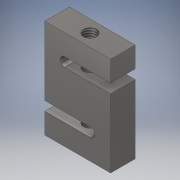
# Autodesk Inventor part: loadcell_s_500kg
Saved by Autodesk Inventor 2019.4 (Build 234330000, 330)
## iProperties
Created: 2020-09-27
Part Number: loadcell_s_500kg
Material: Stainless Steel
Document SubType Name: Modeling
Designer: deanv
Density: 8 g/cm^3
Appearance: Semi-Polished
Author: deanv
Autodesk Inventor part; units mm, degrees
ref_plane "YZ Plane" through (0, 0, 0) normal (1, 0, 0) x (0, 1, 0)
ref_plane "XZ Plane" through (0, 0, 0) normal (0, 1, 0) x (-1, 0, 0)
ref_plane "XY Plane" through (0, 0, 0) normal (0, 0, 1) x (1, 0, 0)
sketch "Sketch1" plane through (0, 0, 0) normal (0, 0, 1) x (1, 0, 0)
  line L0 (-25.4, -38.1) -> (25.4, -38.1) construction
  line L1 (25.4, -38.1) -> (25.4, 38.1) construction
  line L2 (25.4, 38.1) -> (-25.4, 38.1) construction
  line L3 (-25.4, 38.1) -> (-25.4, -38.1) construction
  line L4 (-25.4, -38.1) -> (25.4, 38.1) construction
  line L5 (25.4, -38.1) -> (-25.4, 38.1) construction
  line L6 (25.4, 38.1) -> (-25.4, 38.1) construction
  line L7 (-25.4, 38.1) -> (-25.4, 22.1) construction
  line L8 (-25.4, 22.1) -> (25.4, 22.1) construction
  line L9 (25.4, 22.1) -> (25.4, 38.1) construction
  line L10 (-25.4, -38.1) -> (25.4, -38.1) construction
  line L11 (25.4, -38.1) -> (25.4, -22.1) construction
  line L12 (25.4, -22.1) -> (-25.4, -22.1) construction
  line L13 (-25.4, -22.1) -> (-25.4, -38.1) construction
  line L14 (25.4, -15) -> (-25.4, -15) construction
  line L15 (-25.4, -15) -> (-25.4, 15) construction
  line L16 (-25.4, 15) -> (25.4, 15) construction
  line L17 (25.4, 15) -> (25.4, -15) construction
  line L18 (25.4, -15) -> (-25.4, 15) construction
  line L19 (-25.4, -15) -> (25.4, 15) construction
  line L20 (-25.4, 22.1) -> (-13.4, 22.1) construction
  line L21 (-13.4, 22.1) -> (-13.4, 15) construction
  line L22 (-13.4, 15) -> (-25.4, 15) construction
  line L23 (-25.4, 15) -> (-25.4, 22.1) construction
  line L24 (25.4, -22.1) -> (13.4, -22.1) construction
  line L25 (13.4, -22.1) -> (13.4, -15) construction
  line L26 (13.4, -15) -> (25.4, -15) construction
  line L27 (25.4, -15) -> (25.4, -22.1) construction
  line L28 (-13.4, 15) -> (-6.3, 15) construction
  line L29 (-6.3, 15) -> (-6.3, 22.1) construction
  line L30 (-6.3, 22.1) -> (-13.4, 22.1) construction
  line L31 (-13.4, 22.1) -> (-13.4, 15) construction
  line L32 (13.4, -22.1) -> (6.3, -22.1) construction
  line L33 (6.3, -22.1) -> (6.3, -15) construction
  line L34 (6.3, -15) -> (13.4, -15) construction
  line L35 (13.4, -15) -> (13.4, -22.1) construction
  arc A0 (-9.85, 22.1) -> (-9.85, 15) centre (-9.85, 18.55) ccw construction
  arc A1 (9.85, -22.1) -> (9.85, -15) centre (9.85, -18.55) ccw construction
  line L36 (25.4, 22.1) -> (25.4, 38.1)
  line L37 (25.4, 38.1) -> (-25.4, 38.1)
  line L38 (-25.4, 38.1) -> (-25.4, -15)
  line L39 (-25.4, -15) -> (9.85, -15)
  arc A2 (9.85, -22.1) -> (9.85, -15) centre (9.85, -18.55) ccw
  line L40 (9.85, -22.1) -> (-25.4, -22.1)
  line L41 (-25.4, -22.1) -> (-25.4, -38.1)
  line L42 (-25.4, -38.1) -> (25.4, -38.1)
  line L43 (25.4, -38.1) -> (25.4, 15)
  line L44 (25.4, 15) -> (-9.85, 15)
  arc A3 (-9.85, 22.1) -> (-9.85, 15) centre (-9.85, 18.55) ccw
  line L45 (-9.85, 22.1) -> (25.4, 22.1)
  line L46 (25.4, 38.1) -> (25.4, 22.1)
  line L47 (25.4, 22.1) -> (-9.85, 22.1)
  line L48 (-9.85, 15) -> (25.4, 15)
  line L49 (25.4, 15) -> (25.4, -38.1)
  line L50 (25.4, -38.1) -> (-25.4, -38.1)
  line L51 (-25.4, -38.1) -> (-25.4, -22.1)
  line L52 (-25.4, -22.1) -> (9.85, -22.1)
  line L53 (-25.4, -15) -> (9.85, -15)
  arc A4 (9.85, -22.1) -> (9.85, -15) centre (9.85, -18.55) ccw
  arc A5 (-9.85, 22.1) -> (-9.85, 15) centre (-9.85, 18.55) ccw
  line L54 (-25.4, -15) -> (-25.4, 38.1)
  line L55 (-25.4, 38.1) -> (25.4, 38.1)
  point P0 (0, 0)
  dimension "d0" = 50.8
  dimension "d1" = 76.2
  dimension "d2" = 50.8
  dimension "d3" = 16
  dimension "d4" = 16
  dimension "d5" = 30
  dimension "d6" = 12
  dimension "d7" = 12
  dimension "d8" = 7.1
  dimension "d9" = 7.1
  constraints: 112 end point, 17 parallel, 16 perpendicular, 12 point on circle, 9 midpoint, 8 horizontal, 7 collinear, 7 point on line, 6 centre point, 6 tangent, 1 concentric
  measures "d0" distance of L2.end L1.end
  measures "d1" distance of L1.end L0.end
  measures "d2" distance of L8.end L7.end
  measures "d3" distance between parallel lines of L2 L8
  measures "d4" distance between parallel lines of L0 L12
  measures "d5" distance of L14.end L15.end
  measures "d6" distance of L21.end L22.end
  measures "d7" distance of L25.end L26.end
  measures "d8" distance of L30.end L29.end
  measures "d9" distance of L33.end L34.end
extrude "Extrusion1" add sketch "Sketch1" along normal blind 19
sketch "Sketch2" plane through (-25.4, 38.1, 0) normal (0, 1, 0) x (1, 0, 0)
  line L0 (0, -19) -> (50.8, 0) construction
  line L1 (50.8, -19) -> (0, 0) construction
  point P0 (25.4, 0)
  point P1 (25.4, -9.5)
  constraints: 4 end point, 1 midpoint
hole "Hole1" at (0, 38.1, 9.5) direction (0, -1, 0) diameter 10.106 end through all thread size "M12x1.75" class "6H" standard "ISO Metric profile"
equation "\"d2\" = d0"
equation "\"d4\" = d3"
body "Solid1"
